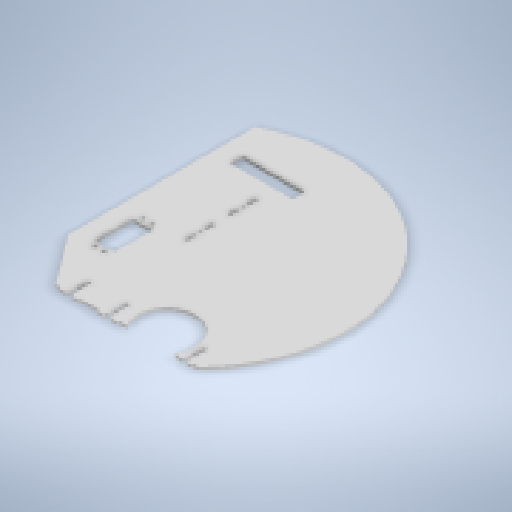
# Autodesk Inventor part: боковые стороны головы
Saved by Autodesk Inventor 2023.2 (Build 272271030, 271C)
## iProperties
Created: 2024-01-31
Part Number: боковые стороны головы
Material: Типовые
Document SubType Name: Modeling
Designer: I9232
Density: 1 g/cm^3
Appearance: По умолчанию
Author: I9232
Autodesk Inventor part; units mm, degrees
ref_plane "YZ Plane" through (0, 0, 0) normal (1, 0, 0) x (0, 1, 0)
ref_plane "XZ Plane" through (0, 0, 0) normal (0, 1, 0) x (-1, 0, 0)
ref_plane "XY Plane" through (0, 0, 0) normal (0, 0, 1) x (1, 0, 0)
sketch "Эскиз1" plane through (0, 0, 0) normal (0, 1, 0) x (-1, 0, 0)
  line L0 (-188.1037, -96.7538) -> (-38.405, -96.7538)
  line L1 (0, -148.7467) -> (0, -343.7987)
  line L2 (-38.405, -96.7538) -> (0, -148.7467)
  arc A0 (-188.1037, -96.7538) -> (0, -343.7987) centre (-75.4996, -206.1503) ccw
  point P0 (0, 0)
  point P1 (-169.7729, -152.9638)
  dimension "d66" = 96.7538
  dimension "d67" = 148.7467
  dimension "d68" = 126.452
  constraints: 6 end point, 2 point on circle, 1 centre point, 1 horizontal, 1 perpendicular, 1 point on line
  measures "d66" distance from line of L0 point (0, 0)
  measures "d67" distance of point (0, 0) L1.start
  measures "d68" angle of L0 L2
extrude "Выдавливание2" add sketch "Эскиз1" along normal blind 3
sketch "Эскиз3" plane through (0, 0, 0) normal (0, -1, 0) x (1, 0, 0)
  circle A0 centre (138.4507, -112.6325) radius 30
  line L0 (146.7814, -112.6325) -> (51.9196, -112.6325) construction
  point P0 (0, 0)
  constraints: 2 end point, 1 centre point, 1 horizontal, 1 point on line
extrude "Выдавливание3" cut sketch "Эскиз3" against normal through all
sketch "Эскиз4" plane through (0, 3, 0) normal (0, 1, 0) x (1, 0, 0)
  line L0 (40, 196.7538) -> (19, 196.7538)
  line L1 (19, 196.7538) -> (19, 156.7538)
  line L2 (19, 156.7538) -> (40, 156.7538)
  line L3 (40, 156.7538) -> (40, 196.7538)
  line L4 (40, 176.7538) -> (19, 176.7538) construction
  circle A0 centre (34.25, 201.9538) radius 2.15
  circle A1 centre (24.75, 201.9538) radius 2.15
  line L5 (0, 343.7987) -> (0, 148.7467) projected
  line L6 (29.5, 196.7538) -> (29.5, 203.7538) construction
  line L7 (39, 207.1538) -> (20, 207.1538) construction
  line L8 (39, 207.1538) -> (39, 196.7538) construction
  line L9 (20, 207.1538) -> (20, 196.7538) construction
  line L10 (34.25, 207.1538) -> (34.25, 196.7538) construction
  line L11 (24.75, 207.1538) -> (24.75, 196.7538) construction
  circle A2 centre (34.25, 151.5538) radius 2.15
  circle A3 centre (24.75, 151.5538) radius 2.15
  point P0 (0, 0)
  point P1 (39, 201.9538)
  dimension "d10" = 40
  dimension "d97" = 7
  dimension "d109" = 21
  dimension "d115" = 9.5
  dimension "d116" = 19
  dimension "d117" = 5.2
  dimension "d118" = 19
  dimension "d119" = 1
  constraints: 22 end point, 6 midpoint, 4 centre point, 4 point on line, 4 symmetric about line, 3 vertical, 2 parallel, 2 perpendicular, 1 horizontal, 2 other
  measures "d10" distance of L0.end L1.end
  measures "d97" distance of L6.start L6.end
  measures "d109" distance of L0.start L0.end
  measures "d115" distance of A1.centre A0.centre
  measures "d116" distance of L7.start L7.end
  measures "d117" distance from line of L0 A0.centre
  measures "d118" distance between parallel lines of L5 L1
  measures "d119" distance from line of L0.end L9
extrude "Выдавливание4" cut sketch "Эскиз4" against normal blind 10
sketch "Эскиз6" plane through (188.1037, 0, -96.7538) normal (0, 0, 1) x (1, 0, 0)
  line L0 (-24.1997, 3) -> (-75.1062, 3) construction
  line L1 (-83.1062, 3) -> (-90.1062, 3)
  line L2 (-90.1062, 3) -> (-90.1062, 0)
  line L3 (-90.1062, 0) -> (-83.1062, 0)
  line L4 (-83.1062, 0) -> (-83.1062, 3)
  line L5 (-97.1062, 3) -> (-104.1062, 3)
  line L6 (-104.1062, 3) -> (-104.1062, 0)
  line L7 (-104.1062, 0) -> (-97.1062, 0)
  line L8 (-97.1062, 0) -> (-97.1062, 3)
  line L9 (-123.1037, 3) -> (-130.1037, 3)
  line L10 (-130.1037, 3) -> (-130.1037, 0)
  line L11 (-130.1037, 0) -> (-123.1037, 0)
  line L12 (-123.1037, 0) -> (-123.1037, 3)
  line L13 (-137.1037, 3) -> (-144.1037, 3)
  line L14 (-144.1037, 3) -> (-144.1037, 0)
  line L15 (-144.1037, 0) -> (-137.1037, 0)
  line L16 (-137.1037, 0) -> (-137.1037, 3)
  line L17 (-188.1037, 0) -> (-75.1062, 0) projected
  line L18 (0, 0) -> (0, 3) projected
  line L19 (-188.1037, 0) -> (-188.1037, 3) projected
  line L20 (-6.1997, 3) -> (-10.1997, 3)
  line L21 (-10.1997, 3) -> (-10.1997, 0)
  line L22 (-10.1997, 0) -> (-6.1997, 0)
  line L23 (-6.1997, 0) -> (-6.1997, 3)
  line L24 (-15.1997, 3) -> (-19.1997, 3)
  line L25 (-19.1997, 3) -> (-19.1997, 0)
  line L26 (-19.1997, 0) -> (-15.1997, 0)
  line L27 (-15.1997, 0) -> (-15.1997, 3)
  line L28 (-24.1997, 3) -> (0, 3) projected
  line L29 (-24.1997, 3) -> (-24.1997, 0) projected
  line L30 (-75.1062, 0) -> (-75.1062, 3) projected
  point P0 (-97.1062, 1.5)
  point P1 (-90.1062, 1.5)
  point P2 (-122.3404, 3.4597)
  point P3 (-137.1037, 1.5)
  point P4 (-130.1037, 1.5)
  point P5 (-126.6037, 0)
  point P6 (-140.6037, 0)
  point P7 (0, 1.5)
  point P8 (-188.1037, 1.5)
  point P9 (-15.1997, 1.5)
  point P10 (-10.1997, 1.5)
  point P11 (2.7481, -1.2329)
  point P12 (2.7481, 1.7671)
  point P13 (-75.1062, 1.5)
  point P14 (-83.1062, 1.5)
  dimension "d20" = 7
  dimension "d21" = 7
  dimension "d22" = 3
  dimension "d23" = 7
  dimension "d24" = 7
  dimension "d25" = 7
  dimension "d26" = 3
  dimension "d27" = 7
  dimension "d28" = 3
  dimension "d50" = 44
  dimension "d75" = 4
  dimension "d76" = 4
  dimension "d77" = 3
  dimension "d79" = 5
  dimension "d80" = 0
  dimension "d81" = 0
  dimension "d82" = 5
  dimension "d91" = 8
  constraints: 48 end point, 13 parallel, 12 midpoint, 6 horizontal, 6 perpendicular, 4 point on line
  measures "d20" distance of L2.end L3.end
  measures "d21" distance of L6.end L7.end
  measures "d22" distance of L7.end L5.start
  measures "d23" distance of point (-97.106, 1.5) point (-90.106, 1.5)
  measures "d24" distance of L10.end L11.end
  measures "d25" distance of L14.end L15.end
  measures "d26" distance of L15.end L13.start
  measures "d27" distance of point (-137.104, 1.5) point (-130.104, 1.5)
  measures "d28" distance of L11.end L9.start
  measures "d50" distance from line of point (-188.104, 1.5) L14
  measures "d75" distance of L21.end L22.end
  measures "d76" distance of L25.end L26.end
  measures "d77" distance of L26.end L24.start
  measures "d79" distance between parallel lines of L27 L21
  measures "d80" distance between parallel lines of L28 L24
  measures "d81" distance between parallel lines of L28 L20
  measures "d82" distance between parallel lines of L29 L25
  measures "d91" distance of point (-75.106, 1.5) point (-83.106, 1.5)
extrude "Выдавливание5" add sketch "Эскиз6" along normal blind 2
sketch "Эскиз7" plane through (0, 0, 0) normal (0, -1, 0) x (1, 0, 0)
  line L0 (51, -96.7538) -> (58, -96.7538) projected
  line L1 (58, -96.7538) -> (51, -96.7538)
  line L2 (54.5, -96.7538) -> (56.25, -96.7538)
  line L3 (56.25, -116.7538) -> (54.5, -116.7538)
  line L4 (54.5, -116.7538) -> (54.5, -96.7538) construction
  line L5 (52.75, -116.7538) -> (54.5, -116.7538)
  line L6 (51.45, -104.8538) -> (51.45, -107.3538)
  line L7 (57.55, -107.3538) -> (57.55, -104.8538)
  line L8 (57.55, -104.8538) -> (51.45, -107.3538) construction
  line L9 (51.45, -104.8538) -> (57.55, -107.3538) construction
  line L10 (54.5, -104.8538) -> (54.5, -106.1038)
  line L11 (57.55, -104.8538) -> (56.25, -104.8538)
  line L12 (52.75, -104.8538) -> (51.45, -104.8538)
  line L13 (51.45, -107.3538) -> (52.75, -107.3538)
  line L14 (56.25, -107.3538) -> (57.55, -107.3538)
  line L15 (56.25, -96.7538) -> (56.25, -104.8538)
  line L16 (56.25, -107.3538) -> (56.25, -116.7538)
  line L17 (52.75, -96.7538) -> (52.75, -104.8538)
  line L18 (52.75, -107.3538) -> (52.75, -116.7538)
  line L19 (97.9975, -96.7538) -> (90.9975, -96.7538)
  line L20 (90.9975, -96.7538) -> (97.9975, -96.7538)
  line L21 (97.9975, -96.7538) -> (90.9975, -96.7538)
  line L22 (94.4975, -96.7538) -> (96.2475, -96.7538)
  line L23 (96.2475, -116.7538) -> (94.4975, -116.7538)
  line L24 (94.4975, -116.7538) -> (94.4975, -96.7538) construction
  line L25 (92.7475, -116.7538) -> (94.4975, -116.7538)
  line L26 (91.4475, -102.7083) -> (91.4475, -105.2083)
  line L27 (97.5475, -105.2083) -> (97.5475, -102.7083)
  line L28 (97.5475, -102.7083) -> (91.4475, -105.2083) construction
  line L29 (91.4475, -102.7083) -> (97.5475, -105.2083) construction
  line L30 (94.4975, -104.8538) -> (94.4975, -103.9583)
  line L31 (97.5475, -102.7083) -> (96.2475, -102.7083)
  line L32 (92.7475, -102.7083) -> (91.4475, -102.7083)
  line L33 (91.4475, -105.2083) -> (92.7475, -105.2083)
  line L34 (96.2475, -105.2083) -> (97.5475, -105.2083)
  line L35 (96.2475, -96.7538) -> (96.2475, -102.7083)
  line L36 (96.2475, -105.2083) -> (96.2475, -116.7538)
  line L37 (92.7475, -96.7538) -> (92.7475, -102.7083)
  line L38 (92.7475, -105.2083) -> (92.7475, -116.7538)
  line L39 (183.8274, -96.7538) -> (166.9805, -96.7538)
  line L40 (166.9805, -96.7538) -> (183.8274, -96.7538)
  line L41 (175.4039, -96.7538) -> (177.1539, -96.7538)
  line L42 (177.1539, -116.7538) -> (175.4039, -116.7538)
  line L43 (175.4039, -116.7538) -> (175.4039, -96.7538) construction
  line L44 (173.6539, -116.7538) -> (175.4039, -116.7538)
  line L45 (172.3539, -104.8538) -> (172.3539, -107.3538)
  line L46 (178.4539, -107.3538) -> (178.4539, -104.8538)
  line L47 (178.4539, -104.8538) -> (172.3539, -107.3538) construction
  line L48 (172.3539, -104.8538) -> (178.4539, -107.3538) construction
  line L49 (175.4039, -104.8538) -> (175.4039, -106.1038)
  line L50 (178.4539, -104.8538) -> (177.1539, -104.8538)
  line L51 (173.6539, -104.8538) -> (172.3539, -104.8538)
  line L52 (172.3539, -107.3538) -> (173.6539, -107.3538)
  line L53 (177.1539, -107.3538) -> (178.4539, -107.3538)
  line L54 (177.1539, -96.7538) -> (177.1539, -104.8538)
  line L55 (177.1539, -107.3538) -> (177.1539, -116.7538)
  line L56 (173.6539, -96.7538) -> (173.6539, -104.8538)
  line L57 (173.6539, -107.3538) -> (173.6539, -116.7538)
  line L58 (172.9039, -96.7538) -> (177.9039, -96.7538) projected
  point P0 (0, 0)
  dimension "d31" = 20
  dimension "d32" = 3.5
  dimension "d33" = 6.1
  dimension "d34" = 2.5
  dimension "d43" = 8.1
  dimension "d51" = 3.5
  dimension "d69" = 20
  dimension "d70" = 3.5
  dimension "d71" = 6.1
  dimension "d72" = 2.5
  dimension "d73" = 8.1
  dimension "d74" = 3.5
  dimension "d83" = 20
  dimension "d84" = 3.5
  dimension "d85" = 6.1
  dimension "d86" = 2.5
  dimension "d87" = 8.1
  dimension "d88" = 3.5
  dimension "d89" = 8.1
  dimension "d90" = 1.3
  constraints: 114 end point, 24 parallel, 13 perpendicular, 11 midpoint, 10 horizontal, 6 collinear, 6 symmetric about line, 3 equal length
  measures "d31" distance of L2.end L3.start
  measures "d32" distance of L5.start L3.start
  measures "d33" distance of L6.end L7.start
  measures "d34" distance of L6.start L6.end
  measures "d43" distance of point (54.5, -96.754) L10.start
  measures "d51" distance between parallel lines of L15 L17
  measures "d69" distance of L22.end L36.end
  measures "d70" distance of L25.start L36.end
  measures "d71" distance of L28.end L27.start
  measures "d72" distance of L29.start L28.end
  measures "d73" distance of point (94.497, -96.754) L30.start
  measures "d74" distance between parallel lines of L35 L37
  measures "d83" distance of L54.start L42.start
  measures "d84" distance of L44.start L42.start
  measures "d85" distance of L47.end L46.start
  measures "d86" distance of L45.start L47.end
  measures "d87" distance of point (175.404, -96.754) L49.start
  measures "d88" distance between parallel lines of L54 L56
  measures "d89" distance of L54.start L54.end
  measures "d90" distance of L53.start L46.start
extrude "Выдавливание6" cut sketch "Эскиз7" against normal blind 3
sketch "Эскиз9" plane through (0, 3, 0) normal (0, 1, 0) x (1, 0, 0)
  line L0 (20.2862, 311.0097) -> (85.7772, 311.0097)
  line L1 (85.7772, 311.0097) -> (85.7772, 298.0323)
  line L2 (85.7772, 298.0323) -> (20.2862, 298.0323)
  line L3 (20.2862, 298.0323) -> (20.2862, 311.0097)
  point P0 (0, 0)
  constraints: 8 end point, 2 parallel, 1 horizontal, 1 perpendicular
extrude "Выдавливание7" cut sketch "Эскиз9" against normal blind 10
sketch "Эскиз10" plane through (0, 0, 0) normal (0, -1, 0) x (1, 0, 0)
  line L0 (68.2886, -269.6013) -> (65.2911, -269.6013) projected
  line L1 (68.2886, -279.6013) -> (68.2886, -269.6013) projected
  line L2 (65.2911, -269.6013) -> (65.2911, -279.6013) projected
  line L3 (65.2911, -279.6013) -> (68.2886, -279.6013) projected
  line L4 (65.2911, -249.6013) -> (65.2911, -259.6013) projected
  line L5 (68.2886, -259.6013) -> (68.2886, -249.6013) projected
  line L6 (65.2911, -259.6013) -> (68.2886, -259.6013) projected
  line L7 (68.2886, -249.6013) -> (65.2911, -249.6013) projected
  line L8 (68.2886, -224.6013) -> (65.2911, -224.6013) projected
  line L9 (68.2886, -234.6013) -> (68.2886, -224.6013) projected
  line L10 (65.2911, -224.6013) -> (65.2911, -234.6013) projected
  line L11 (65.2911, -234.6013) -> (68.2886, -234.6013) projected
  line L12 (65.2911, -214.6013) -> (68.2886, -214.6013) projected
  line L13 (65.2911, -204.6013) -> (65.2911, -214.6013) projected
  line L14 (68.2886, -214.6013) -> (68.2886, -204.6013) projected
  line L15 (68.2886, -204.6013) -> (65.2911, -204.6013) projected
  circle A0 centre (66.7899, -219.6013) radius 1.75
  line L16 (66.7899, -214.6013) -> (66.7899, -224.6013) construction
  line L17 (66.7899, -259.6013) -> (66.7899, -269.6013) construction
  circle A1 centre (66.7899, -264.6013) radius 1.75
  point P0 (0, 0)
  dimension "d124" = 3.5
  constraints: 6 midpoint, 4 end point, 2 centre point, 1 equal radius
  measures "d124" diameter of A0
extrude "Выдавливание8" cut sketch "Эскиз10" against normal blind 3
